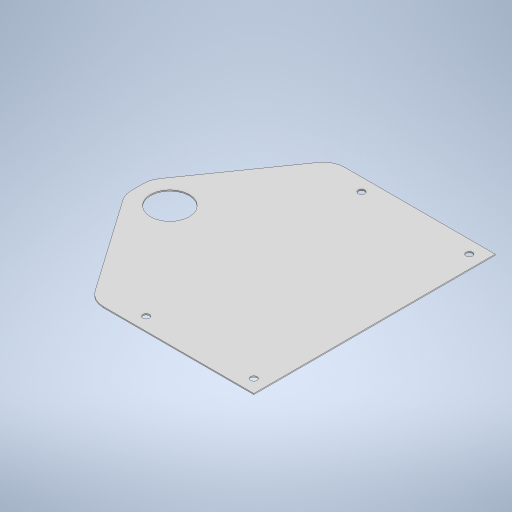
# Autodesk Inventor part: Sketch-3-44
Saved by Autodesk Inventor 2023 (Build 270158000, 158)
## iProperties
Created: 2023-02-21
Part Number: Sketch-3-44
Material: Generic
Document SubType Name: Sheet Metal
Designer: emila
Density: 1 g/cm^3
Appearance: Default
Sheet Metal Rule: Default
Author: emila
Autodesk Inventor part; units mm, degrees
ref_plane "YZ Plane" through (0, 0, 0) normal (1, 0, 0) x (0, 1, 0)
ref_plane "XZ Plane" through (0, 0, 0) normal (0, 1, 0) x (-1, 0, 0)
ref_plane "XY Plane" through (0, 0, 0) normal (0, 0, 1) x (1, 0, 0)
sketch "Sketch2" plane through (0, 0, 0) normal (0, 1, 0) x (-1, 0, 0)
  line L0 (0, 0) -> (69.7934, 0)
  line L1 (110, -53.1522) -> (110, -58.8478)
  line L2 (69.7934, -112) -> (0, -112)
  line L3 (0, -112) -> (0, 0)
  line L4 (77.9858, -4.2654) -> (108.1923, -47.4176)
  line L5 (77.9858, -107.7346) -> (108.1923, -64.5824)
  arc A0 (110, -53.1522) -> (108.1923, -47.4176) centre (100, -53.1522) ccw
  arc A1 (108.1923, -64.5824) -> (110, -58.8478) centre (100, -58.8478) ccw
  arc A2 (77.9858, -4.2654) -> (69.7934, 0) centre (69.7934, -10) ccw
  arc A3 (69.7934, -112) -> (77.9858, -107.7346) centre (69.7934, -102) ccw
  point P0 (110, -112)
  point P1 (110, 0)
  point P2 (75, 0)
  point P3 (110, -50)
  point P4 (75, -112)
  point P5 (110, -62)
  dimension "d10" = 110
  dimension "d11" = 112
  dimension "d34" = 35
  dimension "d35" = 50
  dimension "d36" = 35
  dimension "d37" = 50
  dimension "d38" = 10
  measures "d10" distance of point (110, -112) L2.end
  measures "d11" distance of point (110, 0) point (110, -112)
  measures "d34" distance of point (75, 0) point (110, 0)
  measures "d35" distance of point (110, -50) point (110, 0)
  measures "d36" distance of point (75, -112) point (110, -112)
  measures "d37" distance of point (110, -62) point (110, -112)
  measures "d38" radius of A0
extrude "Plate1" add sketch "Sketch2" along normal blind 0.5
sketch "Sketch3" plane through (0, 0.5, 0) normal (0, 1, 0) x (1, 0, 0)
  line L0 (0, 0) -> (-69.7934, 0) projected
  line L1 (-69.7934, 112) -> (0, 112) projected
  line L2 (0, 112) -> (0, 0) projected
  circle A0 centre (-6, 6) radius 1.55
  line L3 (0, 59.1522) -> (-110, 59.1522) construction
  line L4 (-110, 53.1522) -> (-110, 58.8478) projected
  line L5 (-6, 0) -> (-6, 112) construction
  circle A1 centre (-6, 106) radius 1.55
  circle A2 centre (-56, 6) radius 1.55
  circle A3 centre (-56, 106) radius 1.55
  point P0 (-62, 0)
  point P1 (-62, 112)
  point P2 (-110, 58.8478)
  dimension "d16" = 3.1
  dimension "d17" = 6
  dimension "d18" = 6
  dimension "d21" = 100
  dimension "d24" = 50
  constraints: 4 centre point, 4 end point, 3 point on line, 2 horizontal, 1 perpendicular, 1 vertical, 8 other
  measures "d16" diameter of A0
  measures "d17" distance from line of L0 A0.centre
  measures "d18" distance from line of L2 A0.centre
  measures "d21" distance of A0.centre A1.centre
  measures "d24" distance of A0.centre A2.centre
hole "Hole1" at (-56, 0.5, -6) at (-6, 0.5, -6) at (-6, 0.5, -106) at (-56, 0.5, -106) direction (0, -1, 0) diameter 3.1 end through all
sketch "Sketch4" plane through (0, 0.5, 0) normal (0, 1, 0) x (1, 0, 0)
  circle A0 centre (-56, 6) radius 1.55 projected
  circle A1 centre (-56, 106) radius 1.55 projected
  line L0 (-56, 6) -> (-56, 106) construction
  line L1 (-56, 106) -> (-56, 56)
  line L2 (-56, 56) -> (-110, 56) construction
  line L3 (-110, 53.1522) -> (-110, 58.8478) projected
  circle A2 centre (-95, 56) radius 9
  line L4 (-110, 53.1522) -> (-110, 58.8478) projected
  point P0 (0, 0)
  dimension "d39" = 18
  dimension "d40" = 15
  constraints: 6 end point, 3 midpoint, 1 centre point, 1 point on line
  measures "d39" diameter of A2
  measures "d40" distance of point (-110, 56) A2.centre
hole "Hole2" at (-95, 0.5, -56) direction (0, -1, 0) diameter 18 end through all
equation "\"d32\" = Thickness"
equation "\"d36\" = d34"
equation "\"BendRadius\" = Thickness"
equation "\"BendReliefWidth\" = Thickness"
equation "\"BendReliefDepth\" = 0.5 * Thickness"
equation "\"CornerReliefSize\" = 4 * Thickness"
equation "\"MinimumRemnant\" = 2 * Thickness"
equation "\"TransitionRadius\" = BendRadius"
equation "\"JacobiRadiusSize\" = BendRadius"
equation "\"GapSize\" = Thickness"
body "Solid1"
